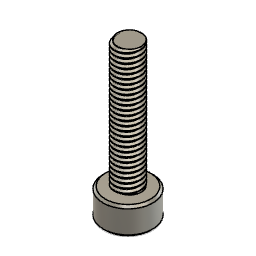
leg-v2-v20 (Autodesk Fusion 360 archive; units mm, degrees)
design "Cub Head Screw HEX (M3, 14mm)"
Autodesk Fusion 360 part; units mm, degrees
sketch "Sketch1" plane through (0, 0, 0) normal (0, 1, 0) x (1, 0, 0)
  circle A0 centre (0, 0) radius 1.5
  circle A1 centre (0, 0) radius 2.75
  line L0 (0.7217, -1.25) -> (1.4434, 0)
  line L1 (1.4434, 0) -> (0.7217, 1.25)
  line L2 (0.7217, 1.25) -> (-0.7217, 1.25)
  line L3 (-0.7217, 1.25) -> (-1.4434, 0)
  line L4 (-1.4434, 0) -> (-0.7217, -1.25)
  line L5 (-0.7217, -1.25) -> (0.7217, -1.25)
  dimension "d6" = 3
  dimension "d7" = 5.5
  dimension "d8" = 1.25
  constraint coincident A0.centre A1.centre
  constraint concentric A0 A1
  measures "d6" diameter of A0
  measures "d7" diameter of A1
  measures "d8" distance of A0.centre L5
extrude "Extrude1" add sketch "Sketch1" along normal blind 3 contours A0 | A1 | L0 L1 L2 L3 L4 L5
extrude "Extrude2" add sketch "Sketch1" along normal blind 17 contours A0 | L0 L1 L2 L3 L4 L5
extrude "Extrude3" cut sketch "Sketch1" along normal blind 1.5 contours L0 L1 L2 L3 L4 L5
thread "Thread1" "ISO Metric profile 3.0 M3x0.5 6g" major diameter 2.927 minor diameter 2.3555 pitch 0.5 angle 60 modelled right hand crest width 0.0713 on face at (1.4925, 7.6667, -0.1494) crest through (1.4635, 2.875, 0)
chamfer "Chamfer2" distance 0.25 angle 45 1 edges at (-2.5639, 3, 0.9944) 1 faces at (-0.0685, 0, 1.7474)
equation "Thread_Diameter = 3 mm"
equation "Thread_Length = 14 mm"
equation "Head_Diameter = 5.5 mm"
equation "Head_Height = 3 mm"
equation "Hex_Size = 2.5 mm"
equation "d6 = Thread_Diameter"
equation "d7 = Head_Diameter"
equation "d8 = Hex_Size / 2"
equation "d9 = Head_Height"
equation "d11 = Head_Height + Thread_Length"
equation "d13 = Head_Height / 2"

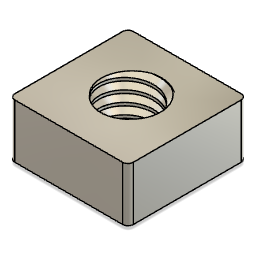
design "Square-Nut (M3)"
Autodesk Fusion 360 part; units mm, degrees
sketch "Sketch1" plane through (0, 0, 0) normal (0, 1, 0) x (1, 0, 0)
  line L0 (2.5, -2.75) -> (-2.5, -2.75)
  line L1 (-2.75, -2.5) -> (-2.75, 2.5)
  line L2 (-2.5, 2.75) -> (2.5, 2.75)
  line L3 (2.75, 2.5) -> (2.75, -2.5)
  line L4 (2.75, -2.75) -> (-2.75, 2.75) construction
  line L5 (-2.75, -2.75) -> (2.75, 2.75) construction
  circle A0 centre (0, 0) radius 1.5
  arc A1 (-2.5, 2.75) -> (-2.75, 2.5) centre (-2.5, 2.5) ccw
  arc A2 (2.75, 2.5) -> (2.5, 2.75) centre (2.5, 2.5) ccw
  arc A3 (2.5, -2.75) -> (2.75, -2.5) centre (2.5, -2.5) ccw
  arc A4 (-2.75, -2.5) -> (-2.5, -2.75) centre (-2.5, -2.5) ccw
  dimension "d1" = 5.5
  dimension "d2" = 5.5
  dimension "d3" = 3
  dimension "d4" = 0.25
  constraint horizontal L0
  constraint perpendicular L0 L1
  constraint parallel L0 L2
  constraint parallel L1 L3
  constraint coincident L4 A0.centre
  constraint coincident L5 A0.centre
  constraint coincident A0.centre origin
  constraint coincident L4.end L1
  constraint coincident L4.end L2
  constraint tangent L1 A1
  constraint tangent L2 A1
  constraint coincident L5.end L2
  constraint coincident L5.end L3
  constraint tangent L2 A2
  constraint tangent L3 A2
  constraint equal A1 A2
  constraint coincident L4.start L3
  constraint coincident L4.start L0
  constraint tangent L3 A3
  constraint tangent L0 A3
  constraint equal A1 A3
  constraint coincident L5.start L0
  constraint coincident L5.start L1
  constraint tangent L0 A4
  constraint tangent L1 A4
  constraint equal A1 A4
  measures "d1" distance of L4.end L5.end
  measures "d2" distance of L5.start L4.end
  measures "d3" diameter of A0
  measures "d4" radius of A1
extrude "Extrude1" add sketch "Sketch1" along normal blind 2.5
thread "Thread1" "ISO Metric profile 3.0 M3x0.5 6H" major diameter 3.086 minor diameter 2.529 pitch 0.5 angle 60 modelled right hand crest width 0.1368 on face at (1.4981, 1.6667, 0.0748) crest through (1.2645, 0.125, 0)
equation "d2 = d1"

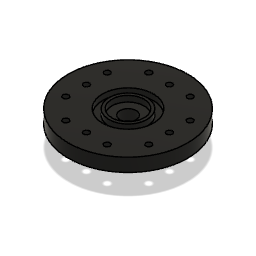
design "MG996R-servo horn"
Autodesk Fusion 360 part; units mm, degrees
sketch "Sketch1" plane through (0, 0, 0) normal (0, 1, 0) x (1, 0, 0)
  circle A0 centre (0, 0) radius 10.35
  circle A1 centre (0, 0) radius 4.4
  circle A2 centre (0, 0) radius 2.8
  circle A3 centre (0, 0) radius 3.3
  circle A4 centre (0, 0) radius 1.4
  circle A5 centre (0, 0) radius 2.6
  circle A6 centre (0, 7.2) radius 0.5
  circle A7 centre (-3.6, 7.2) radius 0.5
  circle A8 centre (3.6, 7.2) radius 0.5
  circle A9 centre (-7.2, 3.6) radius 0.5
  circle A10 centre (-7.2, 0) radius 0.5
  circle A11 centre (-7.2, -3.6) radius 0.5
  circle A12 centre (-3.6, -7.2) radius 0.5
  circle A13 centre (0, -7.2) radius 0.5
  circle A14 centre (3.6, -7.2) radius 0.5
  circle A15 centre (7.2, -3.6) radius 0.5
  circle A16 centre (7.2, 0) radius 0.5
  circle A17 centre (7.2, 3.6) radius 0.5
  dimension "d1" = 20.7
  dimension "d2" = 8.8
  dimension "d3" = 5.6
  dimension "d4" = 6.6
  dimension "d5" = 2.8
  dimension "d6" = 5.2
  dimension "d7" = 1
  dimension "d8" = 7.2
  dimension "d11" = 3.6
  dimension "d12" = 0
  dimension "d14" = 360
  constraint coincident A0.centre A1.centre
  constraint concentric A0 A1
  constraint concentric A0 A2
  constraint concentric A1 A3
  constraint concentric A1 A5
  measures "d1" diameter of A0
  measures "d2" diameter of A1
  measures "d3" diameter of A2
  measures "d4" diameter of A3
  measures "d5" diameter of A4
  measures "d6" diameter of A5
  measures "d7" diameter of A6
  measures "d8" distance of A0.centre A6.centre
extrude "Extrude1" add sketch "Sketch1" against normal blind 3.55 contours A1 | A2 | A3
extrude "Extrude4" add sketch "Sketch1" against normal blind 0.55 contours A5
extrude "Extrude2" add sketch "Sketch1" along normal blind 2.3 contours A0 | A1 | A2 | A3 | A5
extrude "Extrude3" cut sketch "Sketch1" against normal blind 1 from surface at 2.3 contours A1 | A2 | A5
equation "d8 = ( 14.4 / 2 ) * 1 mm"

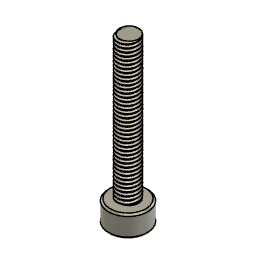
design "Cub Head Screw HEX (M3, 20mm)"
Autodesk Fusion 360 part; units mm, degrees
sketch "Sketch1" plane through (0, 0, 0) normal (0, 1, 0) x (1, 0, 0)
  circle A0 centre (0, 0) radius 1.5
  circle A1 centre (0, 0) radius 2.75
  line L0 (0.7217, -1.25) -> (1.4434, 0)
  line L1 (1.4434, 0) -> (0.7217, 1.25)
  line L2 (0.7217, 1.25) -> (-0.7217, 1.25)
  line L3 (-0.7217, 1.25) -> (-1.4434, 0)
  line L4 (-1.4434, 0) -> (-0.7217, -1.25)
  line L5 (-0.7217, -1.25) -> (0.7217, -1.25)
  dimension "d6" = 3
  dimension "d7" = 5.5
  dimension "d8" = 1.25
  constraint coincident A0.centre A1.centre
  constraint concentric A0 A1
  measures "d6" diameter of A0
  measures "d7" diameter of A1
  measures "d8" distance of A0.centre L5
extrude "Extrude1" add sketch "Sketch1" along normal blind 3 contours A0 | A1 | L0 L1 L2 L3 L4 L5
extrude "Extrude2" add sketch "Sketch1" along normal blind 23 contours A0 | L0 L1 L2 L3 L4 L5
extrude "Extrude3" cut sketch "Sketch1" along normal blind 1.5 contours L0 L1 L2 L3 L4 L5
thread "Thread1" "ISO Metric profile 3.0 M3x0.5 6g" major diameter 2.927 minor diameter 2.3555 pitch 0.5 angle 60 modelled right hand crest width 0.0713 on face at (1.4925, 9.6667, -0.1494) crest through (1.4635, 2.875, 0)
chamfer "Chamfer2" distance 0.25 angle 45 1 edges at (-2.5639, 3, 0.9944) 1 faces at (-0.0685, 0, 1.7474)
equation "Thread_Diameter = 3 mm"
equation "Thread_Length = 20 mm"
equation "Head_Diameter = 5.5 mm"
equation "Head_Height = 3 mm"
equation "Hex_Size = 2.5 mm"
equation "d6 = Thread_Diameter"
equation "d7 = Head_Diameter"
equation "d8 = Hex_Size / 2"
equation "d9 = Head_Height"
equation "d11 = Head_Height + Thread_Length"
equation "d13 = Head_Height / 2"

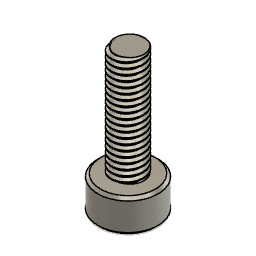
design "Cub Head Screw HEX (M3, 10mm)"
Autodesk Fusion 360 part; units mm, degrees
sketch "Sketch1" plane through (0, 0, 0) normal (0, 1, 0) x (1, 0, 0)
  circle A0 centre (0, 0) radius 1.5
  circle A1 centre (0, 0) radius 2.75
  line L0 (0.7217, -1.25) -> (1.4434, 0)
  line L1 (1.4434, 0) -> (0.7217, 1.25)
  line L2 (0.7217, 1.25) -> (-0.7217, 1.25)
  line L3 (-0.7217, 1.25) -> (-1.4434, 0)
  line L4 (-1.4434, 0) -> (-0.7217, -1.25)
  line L5 (-0.7217, -1.25) -> (0.7217, -1.25)
  dimension "d6" = 3
  dimension "d7" = 5.5
  dimension "d8" = 1.25
  constraint coincident A0.centre A1.centre
  constraint concentric A0 A1
  measures "d6" diameter of A0
  measures "d7" diameter of A1
  measures "d8" distance of A0.centre L5
extrude "Extrude1" add sketch "Sketch1" along normal blind 3 contours A0 | A1 | L0 L1 L2 L3 L4 L5
extrude "Extrude2" add sketch "Sketch1" along normal blind 13 contours A0 | L0 L1 L2 L3 L4 L5
extrude "Extrude3" cut sketch "Sketch1" along normal blind 1.5 contours L0 L1 L2 L3 L4 L5
thread "Thread1" "ISO Metric profile 3.0 M3x0.5 6g" major diameter 2.927 minor diameter 2.3555 pitch 0.5 angle 60 modelled right hand crest width 0.0713 on face at (1.4925, 6.3333, -0.1494) crest through (1.4635, 2.875, 0)
chamfer "Chamfer2" distance 0.25 angle 45 1 edges at (-2.5639, 3, 0.9944) 1 faces at (-0.0685, 0, 1.7474)
equation "Thread_Diameter = 3 mm"
equation "Thread_Length = 10 mm"
equation "Head_Diameter = 5.5 mm"
equation "Head_Height = 3 mm"
equation "Hex_Size = 2.5 mm"
equation "d6 = Thread_Diameter"
equation "d7 = Head_Diameter"
equation "d8 = Hex_Size / 2"
equation "d9 = Head_Height"
equation "d11 = Head_Height + Thread_Length"
equation "d13 = Head_Height / 2"
